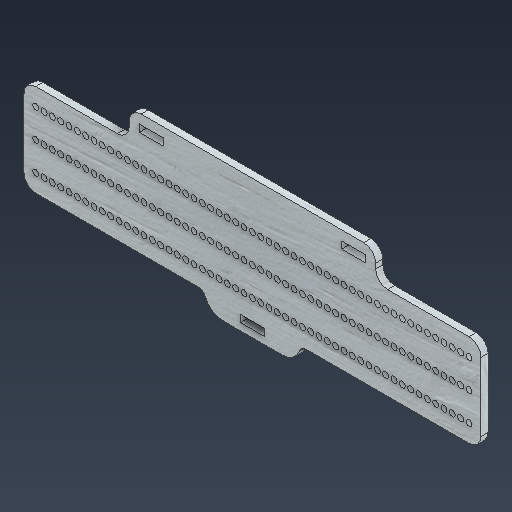
# Autodesk Inventor part: side_frame_revised
Saved by Autodesk Inventor 2025.3 (Build 293356000, 356)
## iProperties
Created: 2025-09-04
Part Number: side_frame_revised
Material: 木材 (楓木)
Document SubType Name: Modeling
Designer: 陳泓任
Density: 0.67 g/cm^3
Appearance: 木材 - 白色刷漆
Mass: 19.0562 g
Surface Area: 249.338 cm^2
Volume: 28.4421 cm^3
Author: 陳泓任
Autodesk Inventor part; units mm, degrees
ref_plane "YZ Plane" through (0, 0, 0) normal (1, 0, 0) x (0, 1, 0)
ref_plane "XZ Plane" through (0, 0, 0) normal (0, 1, 0) x (-1, 0, 0)
ref_plane "XY Plane" through (0, 0, 0) normal (0, 0, 1) x (1, 0, 0)
sketch "草圖1" plane through (0, 0, 0) normal (0, 0, 1) x (1, 0, 0)
  arc A0 (91, -13.3985) -> (96, -8.3985) centre (91, -8.3985) ccw
  arc A1 (-96, -8.3985) -> (-91, -13.3985) centre (-91, -8.3985) ccw
  circle A2 centre (0, 6) radius 1.25
  circle A3 centre (0, -6) radius 1.25
  line L0 (-91, -13.3985) -> (-22.615, -13.3985)
  arc A4 (22.615, -13.3985) -> (19.8099, -15.3349) centre (22.615, -16.3985) ccw
  line L1 (-5, -17.4985) -> (-5, -14.4985)
  line L2 (-5, -14.4985) -> (5, -14.4985)
  line L3 (5, -14.4985) -> (5, -17.4985)
  line L4 (5, -17.4985) -> (-5, -17.4985)
  arc A5 (-19.8099, -15.3349) -> (-22.615, -13.3985) centre (-22.615, -16.3985) ccw
  line L5 (-12.3296, -20.4985) -> (12.3296, -20.4985)
  line L6 (22.615, -13.3985) -> (91, -13.3985)
  line L7 (0, -30.3826) -> (0, 56.5191) construction
  line L8 (-84.6422, 0) -> (139.6626, 0) construction
  line L9 (0, 6) -> (0, -6)
  circle A6 centre (3.5, 6) radius 1.25
  circle A7 centre (3.5, -6) radius 1.25
  circle A8 centre (-3.5, 6) radius 1.25
  circle A9 centre (-3.5, -6) radius 1.25
  circle A10 centre (7, 6) radius 1.25
  circle A11 centre (7, -6) radius 1.25
  circle A12 centre (-7, 6) radius 1.25
  circle A13 centre (-7, -6) radius 1.25
  circle A14 centre (10.5, 6) radius 1.25
  circle A15 centre (10.5, -6) radius 1.25
  circle A16 centre (-10.5, 6) radius 1.25
  circle A17 centre (-10.5, -6) radius 1.25
  circle A18 centre (14, 6) radius 1.25
  circle A19 centre (14, -6) radius 1.25
  circle A20 centre (-14, 6) radius 1.25
  circle A21 centre (-14, -6) radius 1.25
  circle A22 centre (17.5, 6) radius 1.25
  circle A23 centre (17.5, -6) radius 1.25
  circle A24 centre (-17.5, 6) radius 1.25
  circle A25 centre (-17.5, -6) radius 1.25
  circle A26 centre (21, 6) radius 1.25
  circle A27 centre (21, -6) radius 1.25
  circle A28 centre (-21, 6) radius 1.25
  circle A29 centre (-21, -6) radius 1.25
  circle A30 centre (24.5, 6) radius 1.25
  circle A31 centre (24.5, -6) radius 1.25
  circle A32 centre (-24.5, 6) radius 1.25
  circle A33 centre (-24.5, -6) radius 1.25
  circle A34 centre (28, 6) radius 1.25
  circle A35 centre (28, -6) radius 1.25
  circle A36 centre (-28, 6) radius 1.25
  circle A37 centre (-28, -6) radius 1.25
  circle A38 centre (31.5, 6) radius 1.25
  circle A39 centre (31.5, -6) radius 1.25
  circle A40 centre (-31.5, 6) radius 1.25
  circle A41 centre (-31.5, -6) radius 1.25
  circle A42 centre (35, 6) radius 1.25
  circle A43 centre (35, -6) radius 1.25
  circle A44 centre (-35, 6) radius 1.25
  circle A45 centre (-35, -6) radius 1.25
  circle A46 centre (38.5, 6) radius 1.25
  circle A47 centre (38.5, -6) radius 1.25
  circle A48 centre (-38.5, 6) radius 1.25
  circle A49 centre (-38.5, -6) radius 1.25
  circle A50 centre (42, 6) radius 1.25
  circle A51 centre (42, -6) radius 1.25
  circle A52 centre (-42, 6) radius 1.25
  circle A53 centre (-42, -6) radius 1.25
  circle A54 centre (45.5, 6) radius 1.25
  circle A55 centre (45.5, -6) radius 1.25
  circle A56 centre (-45.5, 6) radius 1.25
  circle A57 centre (-45.5, -6) radius 1.25
  circle A58 centre (49, 6) radius 1.25
  circle A59 centre (49, -6) radius 1.25
  circle A60 centre (-49, 6) radius 1.25
  circle A61 centre (-49, -6) radius 1.25
  circle A62 centre (52.5, 6) radius 1.25
  circle A63 centre (52.5, -6) radius 1.25
  circle A64 centre (-52.5, 6) radius 1.25
  circle A65 centre (-52.5, -6) radius 1.25
  circle A66 centre (56, 6) radius 1.25
  circle A67 centre (56, -6) radius 1.25
  circle A68 centre (-56, 6) radius 1.25
  circle A69 centre (-56, -6) radius 1.25
  circle A70 centre (59.5, 6) radius 1.25
  circle A71 centre (59.5, -6) radius 1.25
  circle A72 centre (-59.5, 6) radius 1.25
  circle A73 centre (-59.5, -6) radius 1.25
  circle A74 centre (63, 6) radius 1.25
  circle A75 centre (63, -6) radius 1.25
  circle A76 centre (-63, 6) radius 1.25
  circle A77 centre (-63, -6) radius 1.25
  circle A78 centre (66.5, 6) radius 1.25
  circle A79 centre (66.5, -6) radius 1.25
  circle A80 centre (-66.5, 6) radius 1.25
  circle A81 centre (-66.5, -6) radius 1.25
  circle A82 centre (70, 6) radius 1.25
  circle A83 centre (70, -6) radius 1.25
  circle A84 centre (-70, 6) radius 1.25
  circle A85 centre (-70, -6) radius 1.25
  circle A86 centre (73.5, 6) radius 1.25
  circle A87 centre (73.5, -6) radius 1.25
  circle A88 centre (-73.5, 6) radius 1.25
  circle A89 centre (-73.5, -6) radius 1.25
  line L10 (-46.75, 37.5) -> (46.75, 37.5)
  line L11 (-96, -8.3985) -> (-96, 20.398)
  line L12 (96, 20.398) -> (96, -8.3985)
  arc A90 (-19.8099, -15.3349) -> (-12.3296, -20.4985) centre (-12.3296, -12.4985) ccw
  arc A91 (12.3296, -20.4985) -> (19.8099, -15.3349) centre (12.3296, -12.4985) ccw
  line L13 (-10.7829, -20.4005) -> (9.25, -20.4005) construction
  line L14 (-47.5, 30.5) -> (-47.5, 33.5)
  line L15 (-47.5, 33.5) -> (-37.5, 33.5)
  line L16 (-37.5, 33.5) -> (-37.5, 30.5)
  line L17 (-37.5, 30.5) -> (-47.5, 30.5)
  line L18 (47.5, 33.5) -> (37.5, 33.5)
  line L19 (47.5, 30.5) -> (47.5, 33.5)
  line L20 (37.5, 30.5) -> (47.5, 30.5)
  line L21 (37.5, 33.5) -> (37.5, 30.5)
  line L22 (-91, 25.398) -> (-56.75, 25.398)
  line L23 (-51.75, 30.398) -> (-51.75, 32.5)
  arc A92 (-91, 25.398) -> (-96, 20.398) centre (-91, 20.398) ccw
  arc A93 (-56.75, 25.398) -> (-51.75, 30.398) centre (-56.75, 30.398) ccw
  arc A94 (-46.75, 37.5) -> (-51.75, 32.5) centre (-46.75, 32.5) ccw
  line L24 (91, 25.398) -> (56.75, 25.398)
  line L25 (51.75, 30.398) -> (51.75, 32.5)
  arc A95 (96, 20.398) -> (91, 25.398) centre (91, 20.398) ccw
  arc A96 (51.75, 30.398) -> (56.75, 25.398) centre (56.75, 30.398) ccw
  arc A97 (51.75, 32.5) -> (46.75, 37.5) centre (46.75, 32.5) ccw
  circle A98 centre (77, 6) radius 1.25
  circle A99 centre (77, -6) radius 1.25
  circle A100 centre (-77, 6) radius 1.25
  circle A101 centre (-77, -6) radius 1.25
  circle A102 centre (80.5, 6) radius 1.25
  circle A103 centre (80.5, -6) radius 1.25
  circle A104 centre (-80.5, 6) radius 1.25
  circle A105 centre (-80.5, -6) radius 1.25
  circle A106 centre (84, 6) radius 1.25
  circle A107 centre (84, -6) radius 1.25
  circle A108 centre (-84, 6) radius 1.25
  circle A109 centre (-84, -6) radius 1.25
  circle A110 centre (87.5, 6) radius 1.25
  circle A111 centre (87.5, -6) radius 1.25
  circle A112 centre (-87.5, 6) radius 1.25
  circle A113 centre (-87.5, -6) radius 1.25
  circle A114 centre (91, 6) radius 1.25
  circle A115 centre (91, -6) radius 1.25
  circle A116 centre (-91, 6) radius 1.25
  circle A117 centre (-91, -6) radius 1.25
  circle A118 centre (0, 18) radius 1.25
  circle A119 centre (-3.5, 18) radius 1.25
  circle A120 centre (-10.5, 18) radius 1.25
  circle A121 centre (-7, 18) radius 1.25
  circle A122 centre (3.5, 18) radius 1.25
  circle A123 centre (7, 18) radius 1.25
  circle A124 centre (10.5, 18) radius 1.25
  circle A125 centre (14, 18) radius 1.25
  circle A126 centre (17.5, 18) radius 1.25
  circle A127 centre (21, 18) radius 1.25
  circle A128 centre (24.5, 18) radius 1.25
  circle A129 centre (28, 18) radius 1.25
  circle A130 centre (-14, 18) radius 1.25
  circle A131 centre (-17.5, 18) radius 1.25
  circle A132 centre (-21, 18) radius 1.25
  circle A133 centre (-24.5, 18) radius 1.25
  circle A134 centre (-28, 18) radius 1.25
  circle A135 centre (35, 18) radius 1.25
  circle A136 centre (31.5, 18) radius 1.25
  circle A137 centre (42, 18) radius 1.25
  circle A138 centre (38.5, 18) radius 1.25
  circle A139 centre (-31.5, 18) radius 1.25
  circle A140 centre (-35, 18) radius 1.25
  circle A141 centre (-42, 18) radius 1.25
  circle A142 centre (-45.5, 18) radius 1.25
  circle A143 centre (-38.5, 18) radius 1.25
  circle A144 centre (45.5, 18) radius 1.25
  circle A145 centre (49, 18) radius 1.25
  circle A146 centre (52.5, 18) radius 1.25
  circle A147 centre (56, 18) radius 1.25
  circle A148 centre (-49, 18) radius 1.25
  circle A149 centre (-52.5, 18) radius 1.25
  circle A150 centre (-56, 18) radius 1.25
  circle A151 centre (-70, 18) radius 1.25
  circle A152 centre (-66.5, 18) radius 1.25
  circle A153 centre (-63, 18) radius 1.25
  circle A154 centre (-59.5, 18) radius 1.25
  circle A155 centre (80.5, 18) radius 1.25
  circle A156 centre (77, 18) radius 1.25
  circle A157 centre (73.5, 18) radius 1.25
  circle A158 centre (70, 18) radius 1.25
  circle A159 centre (66.5, 18) radius 1.25
  circle A160 centre (84, 18) radius 1.25
  circle A161 centre (63, 18) radius 1.25
  circle A162 centre (59.5, 18) radius 1.25
  circle A163 centre (-73.5, 18) radius 1.25
  circle A164 centre (-77, 18) radius 1.25
  circle A165 centre (-80.5, 18) radius 1.25
  circle A166 centre (-84, 18) radius 1.25
  circle A167 centre (-87.5, 18) radius 1.25
  circle A168 centre (-91, 18) radius 1.25
  circle A169 centre (87.5, 18) radius 1.25
  circle A170 centre (91, 18) radius 1.25
  point P0 (0, 0)
  point P1 (0, -14.4985)
  point P2 (-96, 25.398)
  point P3 (-51.75, 37.5)
  dimension "d0" = 10
  dimension "d1" = 3
  dimension "d2" = 3
  dimension "d4" = 2.5
  dimension "d12" = 3
  dimension "d29" = 45.23
  dimension "d92" = 3.5
  dimension "d98" = 5
  dimension "d138" = 8
  dimension "d139" = 7.1
  dimension "d141" = 5
  dimension "d147" = 10
  dimension "d148" = 3
  dimension "d149" = 75
  dimension "d150" = 4
  dimension "d152" = 5
  dimension "d153" = 5
  dimension "d166" = 12
  dimension "d167" = 7.3985
  dimension "d225" = 4.25
  dimension "d226" = 192
  dimension "d229" = 12
  dimension "d234" = 5
  dimension "d235" = 7.398
  dimension "d236" = 19.5
  constraints: 171 centre point, 52 end point, 24 point on circle, 16 tangent, 13 symmetric about line, 8 perpendicular, 7 horizontal, 7 point on line, 4 equal radius, 4 vertical, 2 collinear, 1 midpoint, 320 other
  measures "d0" distance of L3.end L1.start
  measures "d1" distance of L1.start L1.end
  measures "d2" distance between parallel lines of L5 L4
  measures "d4" diameter of A2
  measures "d12" radius of A5
  measures "d29" distance of A4.centre A5.centre
  measures "d92" distance of L9.start A6.centre
  measures "d98" radius of A1
  measures "d138" radius of A90
  measures "d139" distance between parallel lines of L0 L5
  measures "d141" radius of A0
  measures "d147" distance of L17.start L14.start
  measures "d148" distance of L14.start L15.start
  measures "d149" diameter of L16 L7
  measures "d150" distance between parallel lines of L10 L15
  measures "d152" radius of A92
  measures "d153" radius of A93
  measures "d166" distance of L9.end L9.start
  measures "d167" distance from line of L6 A67.centre
  measures "d225" distance between parallel lines of L25 L19
  measures "d226" distance between parallel lines of L12 L11
  measures "d229" distance of L9.start A118.centre
  measures "d234" distance from line of L11 A116.centre
  measures "d235" distance from line of L22 A163.centre
  measures "d236" distance from line of L10 A119.centre
extrude "擠出1" add sketch "草圖1" along normal mid plane 3
sketch "草圖3" plane through (0, 0, 1.5) normal (0, 0, 1) x (1, 0, 0)
  line L0 (0, 52.3829) -> (0, -39.0235)
  line L1 (-112.5881, 0) -> (123.4866, 0)
  line L2 (-19.4643, 23.5445) -> (19.2445, 23.5445)
  line L3 (19.2445, 23.5445) -> (19.2445, -11.2117)
  line L4 (19.2445, -11.2117) -> (-19.4643, -11.2117)
  line L5 (-19.4643, -11.2117) -> (-19.4643, 23.5445)
  circle A0 centre (-17.5, 19.5) radius 1.25 projected
  circle A1 centre (17.5, 19.5) radius 1.25 projected
  point P0 (0, 0)
  point P1 (18.75, 19.5)
  point P2 (-18.75, 19.5)
  dimension "d209" = 34.7562
  dimension "d210" = 22.4234
  constraints: 12 end point, 2 horizontal, 2 parallel, 2 point on line, 1 perpendicular, 1 vertical
  measures "d209" distance of L4.end L2.start
  measures "d210" diameter of L4 L1
